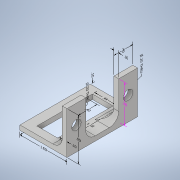
# Autodesk Inventor part: Actobotics Power Switch Mount v2
Saved by Autodesk Inventor 2020 (Build 240168000, 168)
## iProperties
Created: 2019-12-11
Part Number: Actobotics Power Switch Mount v2
Material: Generic
Document SubType Name: Modeling
Designer: AOFUser
Density: 1 g/cm^3
Appearance: Default
Author: AOFUser
Autodesk Inventor part; units mm, degrees
ref_plane "YZ Plane" through (0, 0, 0) normal (1, 0, 0) x (0, 1, 0)
ref_plane "XZ Plane" through (0, 0, 0) normal (0, 1, 0) x (-1, 0, 0)
ref_plane "XY Plane" through (0, 0, 0) normal (0, 0, 1) x (1, 0, 0)
sketch "Sketch1" plane through (0, 0, 0) normal (0, 1, 0) x (-1, 0, 0)
  line L0 (0, 0) -> (-25.4, 0)
  line L1 (-25.4, 0) -> (-25.4, -38.1)
  line L2 (-25.4, -38.1) -> (0, -38.1)
  line L3 (0, -38.1) -> (0, 0)
  dimension "d0" = 25.4
  dimension "d1" = 38.1
  constraints: 8 end point, 2 parallel, 1 horizontal, 1 perpendicular
  measures "d0" distance of L2.end L1.end
  measures "d1" distance of L1.end L0.end
extrude "Extrusion1" add sketch "Sketch1" along normal blind 2.54
sketch "Sketch3" plane through (0, 2.54, 0) normal (0, 1, 0) x (1, 0, 0)
  line L0 (0, 0) -> (5.08, 0)
  line L1 (5.08, 0) -> (5.08, 4.064)
  line L2 (5.08, 4.064) -> (0, 4.064)
  line L3 (0, 4.064) -> (0, 0)
  line L4 (25.4, 38.1) -> (0, 38.1) projected
  line L5 (0, 38.1) -> (5.08, 38.1)
  line L6 (5.08, 38.1) -> (5.08, 34.036)
  line L7 (5.08, 34.036) -> (0, 34.036)
  line L8 (0, 34.036) -> (0, 38.1)
  line L9 (5.08, 4.064) -> (16.256, 4.064)
  line L10 (16.256, 4.064) -> (16.256, 34.036)
  line L11 (16.256, 34.036) -> (5.08, 34.036)
  line L12 (5.08, 34.036) -> (5.08, 4.064)
  dimension "d7" = 5.08
  dimension "d8" = 4.064
  dimension "d9" = 5.08
  dimension "d10" = 4.064
  dimension "d11" = 11.176
  constraints: 24 end point, 6 parallel, 3 horizontal, 3 perpendicular, 1 point on line
  measures "d7" distance of L2.end L1.end
  measures "d8" distance of L1.end L0.end
  measures "d9" distance of L6.end L7.end
  measures "d10" distance of L5.end L6.end
  measures "d11" distance of L11.end L10.end
extrude "Extrusion2" cut sketch "Sketch3" against normal blind 2.54 contours L12 L11 L10 L9
sketch "Sketch4" plane through (0, 2.54, 0) normal (0, 1, 0) x (1, 0, 0)
  line L0 (25.4, 0) -> (25.4, 38.1) projected
  line L1 (25.4, 0) -> (22.86, 0)
  line L2 (22.86, 0) -> (22.86, 10.16)
  line L3 (22.86, 10.16) -> (25.4, 10.16)
  line L4 (25.4, 10.16) -> (25.4, 0)
  line L5 (25.4, 38.1) -> (22.86, 38.1)
  line L6 (22.86, 38.1) -> (22.86, 27.94)
  line L7 (22.86, 27.94) -> (25.4, 27.94)
  line L8 (25.4, 27.94) -> (25.4, 38.1)
  point P0 (0, 0)
  dimension "d14" = 2.54
  dimension "d15" = 10.16
  dimension "d16" = 2.54
  dimension "d17" = 10.16
  constraints: 16 end point, 4 parallel, 2 horizontal, 2 perpendicular
  measures "d14" distance of L2.end L3.end
  measures "d15" distance of L1.end L2.end
  measures "d16" distance of L7.end L6.end
  measures "d17" distance of L6.end L5.end
extrude "Extrusion3" add sketch "Sketch4" along normal blind 20.32
sketch "Sketch5" plane through (22.86, 2.54, -10.16) normal (-1, 0, 0) x (0, 0, 1)
  line L0 (10.16, 20.32) -> (0, 20.32) projected
  line L1 (5.08, 20.32) -> (5.08, 10.16)
  point P0 (10.16, -2.54)
  dimension "d20" = 10.16
  constraints: 2 end point, 1 midpoint, 1 vertical
  measures "d20" distance of L1.start L1.end
hole "Hole1" at (22.86, 12.7, -5.08) direction (1, 0, 0) diameter 5.08 end through all
sketch "Sketch6" plane through (22.86, 2.54, -38.1) normal (-1, 0, 0) x (0, 0, 1)
  line L0 (10.16, 20.32) -> (0, 20.32) projected
  line L1 (5.08, 20.32) -> (5.08, 10.16)
  point P0 (38.1, -2.54)
  dimension "d28" = 10.16
  constraints: 2 end point, 1 midpoint, 1 vertical
  measures "d28" distance of L1.start L1.end
hole "Hole2" at (22.86, 12.7, -33.02) direction (1, 0, 0) diameter 5.08 end through all
fillet "Fillet1" radius 5.08 4 edges at (22.86, 2.54, -5.08) (22.86, 2.54, -33.02) (24.13, 2.54, -27.94) (24.13, 2.54, -10.16)
body "Solid1"
